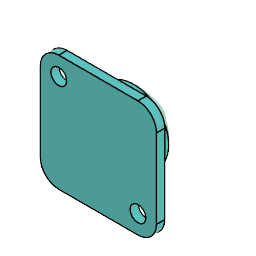
MARS Micromouse (Autodesk Fusion 360 archive; units mm, degrees)
design "Caster Ball"
Autodesk Fusion 360 part; units mm, degrees
sketch "Sketch1" plane through (0, 0, 0) normal (0, 1, 0) x (1, 0, 0)
  line L0 (12.55, -12.55) -> (-12.55, -12.55)
  line L1 (-12.55, -12.55) -> (-12.55, 12.55)
  line L2 (-12.55, 12.55) -> (12.55, 12.55)
  line L3 (12.55, 12.55) -> (12.55, -12.55)
  line L4 (12.55, -12.55) -> (-12.55, 12.55) construction
  line L5 (-12.55, -12.55) -> (12.55, 12.55) construction
  dimension "d1" = 25.1
  constraint horizontal L0
  constraint perpendicular L0 L1
  constraint parallel L0 L2
  constraint parallel L1 L3
  constraint coincident L4 origin
  constraint coincident L5 origin
  constraint equal L0 L1
  measures "d1" distance of L0.end L1.end
extrude "Extrude1" add sketch "Sketch1" along normal blind 1.8
fillet "Fillet1" radius 4 4 edges at (12.55, 0.9, 12.55) (-12.55, 0.9, 12.55) (12.55, 0.9, -12.55) (-12.55, 0.9, -12.55)
sketch "Sketch2" plane through (0, 0, 0) normal (0, 1, 0) x (1, 0, 0)
  arc A0 (-8.55, 12.55) -> (-12.55, 8.55) centre (-8.55, 8.55) ccw
  line L0 (-8.55, 12.55) -> (8.55, 12.55)
  arc A1 (12.55, 8.55) -> (8.55, 12.55) centre (8.55, 8.55) ccw
  line L1 (12.55, 8.55) -> (12.55, -8.55)
  arc A2 (8.55, -12.55) -> (12.55, -8.55) centre (8.55, -8.55) ccw
  line L2 (8.55, -12.55) -> (-8.55, -12.55)
  arc A3 (-12.55, -8.55) -> (-8.55, -12.55) centre (-8.55, -8.55) ccw
  line L3 (-12.55, -8.55) -> (-12.55, 8.55)
  circle A4 centre (-8.55, -8.55) radius 1.7
  circle A5 centre (8.55, 8.55) radius 1.7
  dimension "d6" = 3.4
  dimension "d7" = 3.4
  constraint concentric A3 A4
  constraint concentric A1 A5
  measures "d6" diameter of A4
  measures "d7" diameter of A5
extrude "Extrude2" cut sketch "Sketch2" along normal up to surface (1.8 mm away) contours A4 | A5
sketch "Sketch3" plane through (0, 0, 0) normal (0, 0, 1) x (1, 0, 0)
  line L0 (8.55, 1.8) -> (-8.55, 1.8)
  line L1 (7.6, 1.8) -> (7.6, 7.6)
  circle A0 centre (0, 2.14) radius 9.358
  line L2 (0, 0) -> (0, 12.8)
  line L3 (-7.6, 1.8) -> (-7.6, 7.6)
  circle A1 centre (0, 8.0636) radius 4.7364
  point P0 (4, 10.6)
  point P1 (-4, 10.6)
  point P2 (0, 12.8)
  dimension "d10" = 15.2
  dimension "d11" = 5.8
  dimension "d12" = 8
  dimension "d13" = 3
  dimension "d14" = 11
  constraint coincident L0 L1.start
  constraint perpendicular L0 L1
  constraint coincident L1.end A0
  constraint coincident L2.start origin
  constraint vertical L2
  constraint symmetric L1.start L2 L3.start
  constraint symmetric L1.end L2 L3.end
  constraint coincident A0 P0
  constraint coincident A1 P0
  constraint coincident A0 P1
  constraint coincident A1 P1
  constraint horizontal P0 P1
  constraint coincident A0 L3.end
  constraint coincident A1 P2
  constraint vertical A1.centre P2
  constraint coincident P2 L2.end
  measures "d10" distance of L1 L3
  measures "d11" distance of L3.start L3.end
  measures "d12" distance of P0 P1
  measures "d13" vertical distance of L3.end P1
  measures "d14" distance of L0 P2
revolve "Revolve1" add sketch "Sketch3" angle 360 about axis through (0, 0, 0) along (0, 1, 0) contours L0 L1 A0 L2 A1 | A0 L2 A1 | A0 L2 A1 picked at (1.3111, 8.9913) picked at (0.6836, 11.882)

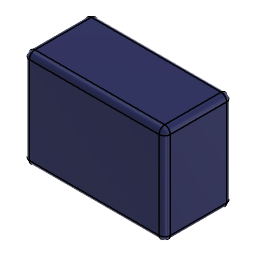
design "Battery"
Autodesk Fusion 360 part; units mm, degrees
sketch "Sketch1" plane through (0, 0, 0) normal (0, 1, 0) x (1, 0, 0)
  line L0 (25, -17.5) -> (-25, -17.5)
  line L1 (-25, -17.5) -> (-25, 17.5)
  line L2 (-25, 17.5) -> (25, 17.5)
  line L3 (25, 17.5) -> (25, -17.5)
  line L4 (25, -17.5) -> (-25, 17.5) construction
  line L5 (-25, -17.5) -> (25, 17.5) construction
  dimension "d1" = 50
  dimension "d2" = 35
  constraint horizontal L0
  constraint perpendicular L0 L1
  constraint parallel L0 L2
  constraint parallel L1 L3
  constraint coincident L4 origin
  constraint coincident L5 origin
  measures "d1" distance of L1.end L2.end
  measures "d2" distance of L0.end L1.end
extrude "Extrude1" add sketch "Sketch1" along normal mid plane 24
fillet "Fillet1" radius 2 12 edges at (0, -12, 17.5) (25, 12, 0) (25, 0, 17.5) (-25, 0, -17.5) (-25, 0, 17.5) (0, 12, -17.5) (0, 12, 17.5) (-25, 12, 0) (25, 0, -17.5) (0, -12, -17.5) (-25, -12, 0) (25, -12, 0) 6 faces at (-25, -4, 5.8333) (-8.3333, -4, -17.5) (8.3333, 12, 5.8333) (8.3333, -12, 5.8333) (25, 4, 5.8333) (-8.3333, 4, 17.5)
